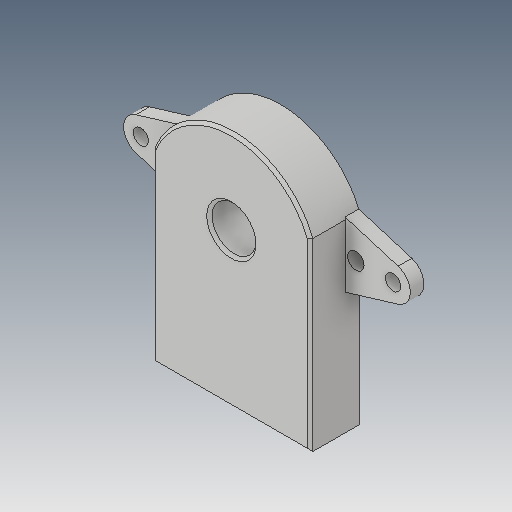
# Autodesk Inventor part: AMT102-1
Saved by Autodesk Inventor 2020.3 (Build 243373000, 373)
## iProperties
Part Number: AMT102-1
Material: 一般
Document SubType Name: Modeling
Designer: highs
Density: 1 g/cm^3
Appearance: 既定
Description: https://www.digikey.jp/product-detail/ja/cui-devices/AMT102-V/102-1307-ND/827015
Stock Number: AMT102-V
Author: highs
Revision Number: "アクセサリが必要らしい． https://www.digikey.jp/product-detail/ja/cui-devices/AMT-8MM/AMT-8MM-ND/4376597"
Autodesk Inventor part; units mm, degrees
ref_plane "YZ Plane" through (0, 0, 0) normal (1, 0, 0) x (0, 1, 0)
ref_plane "XZ Plane" through (0, 0, 0) normal (0, 1, 0) x (-1, 0, 0)
ref_plane "XY Plane" through (0, 0, 0) normal (0, 0, 1) x (1, 0, 0)
sketch "スケッチ1" plane through (0, 0, 0) normal (0, 0, 1) x (1, 0, 0)
  line L0 (0, 0) -> (14.385, 0)
  line L1 (14.385, 0) -> (14.385, 22.14)
  line L2 (14.385, 22.14) -> (23.9245, 25.0353)
  line L3 (23.9245, 31.0447) -> (14.2486, 33.9814)
  line L4 (0, 0) -> (0, 43.38) construction
  arc A0 (14.2486, 33.9814) -> (0, 43.38) centre (0, 27.88) ccw
  circle A1 centre (0, 28.04) radius 4 construction
  line L5 (0, 28.04) -> (33.824, 28.04) construction
  circle A2 centre (16.215, 28.04) radius 1.5
  circle A3 centre (23.0125, 28.04) radius 1.39
  arc A4 (23.9245, 25.0353) -> (23.9245, 31.0447) centre (23.0125, 28.04) ccw
  line L6 (0, 0) -> (-14.385, 0)
  line L7 (-14.385, 0) -> (-14.385, 22.14)
  line L8 (-14.385, 22.14) -> (-23.9245, 25.0353)
  line L9 (-23.9245, 31.0447) -> (-14.2486, 33.9814)
  arc A5 (0, 43.38) -> (-14.2486, 33.9814) centre (0, 27.88) ccw
  circle A6 centre (-16.215, 28.04) radius 1.5
  circle A7 centre (-23.0125, 28.04) radius 1.39
  arc A8 (-23.9245, 31.0447) -> (-23.9245, 25.0353) centre (-23.0125, 28.04) ccw
  dimension "d0" = 15.5
  dimension "d1" = 43.38
  dimension "d2" = 15.34
  dimension "d3" = 8
  dimension "d4" = 14.385
  dimension "d5" = 5.9
  dimension "d6" = 2.78
  dimension "d7" = 3
  dimension "d8" = 16.215
  dimension "d9" = 23.0125
  dimension "d12" = 3.14
  constraints: 20 end point, 9 centre point, 8 point on circle, 8 symmetric about line, 6 point on line, 2 coincident, 2 horizontal, 2 tangent, 1 perpendicular, 1 vertical, 4 other
  measures "d0" radius of A0
  measures "d1" distance of L0.start L4.end
  measures "d2" distance of L5.start L4.end
  measures "d3" diameter of A1
  measures "d4" distance between parallel lines of L4 L1
  measures "d5" distance from line of L1.end L5
  measures "d6" diameter of A3
  measures "d7" diameter of A2
  measures "d8" distance from line of L4 A2.centre
  measures "d9" distance from line of L4 A3.centre
  measures "d12" radius of A4
extrude "押し出し1" add sketch "スケッチ1" along normal blind 2.5
sketch "スケッチ4" plane through (0, 0, 2.5) normal (0, 0, 1) x (1, 0, 0)
  line L0 (-14.385, 0) -> (14.385, 0) projected
  line L1 (-14.385, 0) -> (14.385, 0)
  line L2 (14.385, 0) -> (14.385, 33.6525)
  arc A0 (14.2486, 33.9814) -> (-14.2486, 33.9814) centre (0, 27.88) ccw projected
  arc A1 (14.385, 33.6525) -> (-14.385, 33.6525) centre (0, 27.88) ccw
  line L3 (-14.385, 0) -> (-14.385, 33.6525)
  point P0 (0, 0)
  constraints: 6 end point, 2 point on circle, 1 centre point, 1 coincident, 1 collinear, 1 concentric, 1 perpendicular, 1 vertical
extrude "押し出し3" add sketch "スケッチ4" along normal blind 6.5
sketch "スケッチ5" plane through (0, 0, 9) normal (0, 0, 1) x (1, 0, 0)
  line L0 (0, 0) -> (0, 28.04) construction
  circle A0 centre (0, 28.04) radius 4
  arc A1 (14.2486, 33.9814) -> (-14.2486, 33.9814) centre (0, 27.88) ccw construction
  point P0 (0, 43.38)
  dimension "d20" = 15.34
  dimension "d21" = 8
  constraints: 2 end point, 2 point on circle, 1 centre point, 1 coincident, 1 vertical
  measures "d20" distance of A0.centre point (0, 43.38)
  measures "d21" diameter of A0
extrude "押し出し4" cut sketch "スケッチ5" against normal up to next
chamfer "面取り1" distance 0.5 angle 45 5 edges at (-14.385, 16.8263, 9) (0, 0, 9) (14.385, 16.8263, 9) (0, 43.38, 9) (-4, 28.04, 9)
